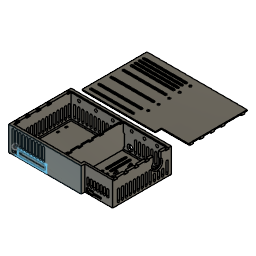
SKRMiniBox CNC (Autodesk Fusion 360 design; units mm, degrees)
part number: 2025-08-04-01-21-32-688
Autodesk Fusion 360 part; units mm, degrees
(part 1 of 2)
other "Base Mesh Feature1"
other "Modify1"
sketch "Sketch2" plane through (0, 0, 0) normal (0, 0, 1) x (1, 0, 0)
  line L0 (-173.9436, -72.9826) -> (-173.9268, 62.9979)
  line L1 (-173.9268, 62.9979) -> (52.0199, 63.0011)
  line L2 (52.0199, 63.0011) -> (52.0199, -64.6029)
  circle A0 centre (28.2811, 19.6527) radius 3.024
  circle A1 centre (-6.7121, 37.2637) radius 3.024
  circle A2 centre (28.2811, 19.6527) radius 3.024
  circle A3 centre (-9.3669, 5.4726) radius 3.024
  circle A4 centre (28.249, -42.7358) radius 3.024
  circle A5 centre (-36.2541, -58.894) radius 3.024
  line L3 (-180, 69) -> (58, 69)
  line L4 (58, 69) -> (58, -70.5015)
  line L5 (-8.0005, -79) -> (-180, -79)
  line L6 (-180, -79) -> (-180, 69)
  arc A6 (47.0198, 63.0011) -> (52.0199, 58.0011) centre (47.0199, 58.0011) ccw
  arc A7 (-168.9436, -72.9826) -> (-173.943, -67.982) centre (-168.943, -67.9826) ccw
  arc A8 (-173.9274, 57.9986) -> (-168.9275, 62.998) centre (-168.9274, 57.998) ccw
  line L7 (-163, 45) -> (-53, 45)
  line L8 (-53, 45) -> (-53, 40)
  line L9 (-53, 40) -> (-163, 40)
  line L10 (-163, 40) -> (-163, 45)
  line L11 (-163, 25) -> (-53, 25)
  line L12 (-53, 25) -> (-53, 20)
  line L13 (-53, 20) -> (-163, 20)
  line L14 (-163, 20) -> (-163, 25)
  line L15 (-163, 57) -> (-53, 57)
  line L16 (-53, 57) -> (-53, -23)
  line L17 (-53, -23) -> (-163, -23)
  line L18 (-163, -23) -> (-163, 57)
  line L19 (-163, -23) -> (-133, -23)
  line L20 (-133, -23) -> (-133, -73)
  line L21 (-133, -73) -> (-163, -73)
  line L22 (-163, -73) -> (-163, -23)
  line L23 (-13.9959, -72.9826) -> (-173.9436, -72.9826)
  line L24 (52.0199, -64.6029) -> (-14, -64.6029)
  line L25 (58, -70.5015) -> (-7.9998, -70.5015)
  line L26 (-13.9959, -72.9826) -> (-13.9959, -64.6029)
  line L27 (-11, -64.5017) -> (-11, -64.5)
  line L28 (-7.9998, -70.5015) -> (-8.0005, -79)
  arc A9 (52.0199, -59.6029) -> (47.0199, -64.6029) centre (47.0199, -59.6029) ccw
  line L29 (-53, 45) -> (-50, 45)
  line L30 (-50, 45) -> (-50, 40)
  line L31 (-50, 40) -> (-53, 40)
  line L32 (-53, 40) -> (-53, 45)
  line L33 (-163, 45) -> (-166, 45)
  line L34 (-166, 45) -> (-166, 40)
  line L35 (-166, 40) -> (-163, 40)
  line L36 (-163, 40) -> (-163, 45)
  line L37 (-53, 25) -> (-50, 25)
  line L38 (-50, 25) -> (-50, 20)
  line L39 (-50, 20) -> (-53, 20)
  line L40 (-53, 20) -> (-53, 25)
  line L41 (-163, 25) -> (-166, 25)
  line L42 (-166, 25) -> (-166, 20)
  line L43 (-166, 20) -> (-163, 20)
  line L44 (-163, 20) -> (-163, 25)
  line L45 (-133, -35) -> (-50, -35)
  line L46 (-50, -35) -> (-50, -40)
  line L47 (-50, -40) -> (-133, -40)
  line L48 (-133, -40) -> (-133, -35)
  line L49 (-163, -35) -> (-166, -35)
  line L50 (-166, -35) -> (-166, -40)
  line L51 (-166, -40) -> (-163, -40)
  line L52 (-163, -40) -> (-163, -35)
  line L53 (-133, -50) -> (-50, -50)
  line L54 (-50, -50) -> (-50, -55)
  line L55 (-50, -55) -> (-133, -55)
  line L56 (-133, -55) -> (-133, -50)
  line L57 (-163, -50) -> (-166, -50)
  line L58 (-166, -50) -> (-166, -55)
  line L59 (-166, -55) -> (-163, -55)
  line L60 (-163, -55) -> (-163, -50)
  line L61 (-133, -65) -> (-50, -65)
  line L62 (-50, -65) -> (-50, -70)
  line L63 (-50, -70) -> (-133, -70)
  line L64 (-133, -70) -> (-133, -65)
  line L65 (-163, -65) -> (-166, -65)
  line L66 (-166, -65) -> (-166, -70)
  line L67 (-166, -70) -> (-163, -70)
  line L68 (-163, -70) -> (-163, -65)
  dimension "d1" = 5
  dimension "d3" = 5
  dimension "d4" = 5
  dimension "d5" = 80
  dimension "d6" = 30
  dimension "d7" = 50
  dimension "d8" = 5
  constraint tangent L1 A6
  constraint tangent L2 A6
  constraint tangent L1 A8
  constraint tangent L0 A8
  constraint tangent L0 A7
  constraint horizontal L3
  constraint vertical L4
  constraint horizontal L5
  constraint vertical L6
  constraint coincident L2 A6.end
  constraint coincident L1 A6.start
  constraint coincident L0 A7.end
  constraint coincident L1 A8.end
  constraint coincident L0 A8.start
  constraint horizontal L7
  constraint vertical L8
  constraint horizontal L9
  constraint vertical L10
  constraint horizontal L11
  constraint vertical L12
  constraint horizontal L13
  constraint vertical L14
  constraint horizontal L15
  constraint vertical L16
  constraint horizontal L17
  constraint vertical L18
  constraint horizontal L19
  constraint vertical L20
  constraint horizontal L21
  constraint vertical L22
  constraint vertical L2
  constraint perpendicular L23 L26
  constraint coincident L24 L26.end
  constraint perpendicular L24 L26
  constraint tangent L2 A9
  constraint tangent L24 A9
  constraint coincident L24 A9.end
  constraint coincident L2 A9.start
  constraint tangent A7 L23
  constraint horizontal L29
  constraint vertical L30
  constraint horizontal L31
  constraint vertical L32
  constraint horizontal L33
  constraint vertical L34
  constraint horizontal L35
  constraint vertical L36
  constraint horizontal L37
  constraint vertical L38
  constraint horizontal L39
  constraint vertical L40
  constraint horizontal L41
  constraint vertical L42
  constraint horizontal L43
  constraint vertical L44
  constraint horizontal L45
  constraint vertical L46
  constraint horizontal L47
  constraint vertical L48
  constraint coincident L20 L45.start
  constraint horizontal L49
  constraint vertical L50
  constraint horizontal L51
  constraint vertical L52
  constraint coincident L22 L49.start
  constraint horizontal L53
  constraint vertical L54
  constraint horizontal L55
  constraint vertical L56
  constraint coincident L20 L53.start
  constraint horizontal L57
  constraint vertical L58
  constraint horizontal L59
  constraint vertical L60
  constraint coincident L22 L57.start
  constraint horizontal L61
  constraint vertical L62
  constraint horizontal L63
  constraint vertical L64
  constraint coincident L20 L61.start
  constraint horizontal L65
  constraint vertical L66
  constraint horizontal L67
  constraint vertical L68
  constraint coincident L22 L65.start
  measures "d1" radius of A6
  measures "d3" radius of A8
  measures "d4" radius of A7
  measures "d5" distance of L15.start L17.end
  measures "d6" distance of L17.end L19.end
  measures "d7" distance of L17.end L21.end
  measures "d8" radius of A9
extrude "Extrude1" add sketch "Sketch2" along normal blind 2 contours L0 A7 L23 L65 L66 L67 | L0 L1 L2 A6 A7 A8 L15 L16 L17 L18 L20 L22 L23 L24 L26 A9 L29 L30 L31 L33 L34 L35 L37 L38 L39 L41 L42 L43 L45 L46 L47 L49 L50 L51 L53 L54 L55 L57 L58 L59 L61 L62 L63 L65 | A7 L22 L23 L67 | L0 L1 A8 | A7 L22 L65 L67 L68 | A7 L65 L66 L67 | L20 L21 L22 L23 | L17 L19 L20 L22 L23 L48 L52 L56 L60 L64 L68 | L1 L2 A6 | L22 L57 L58 L59 L60 | L20 L61 L62 L63 L64 | L2 L24 A9 | L22 L49 L50 L51 L52 | L20 L53 L54 L55 L56 | L13 L16 L17 L18 L19 | L20 L45 L46 L47 L48 | L11 L12 L13 L14 L16 L18 L40 L44 | L14 L18 L41 L42 L43 L44 | L12 L16 L37 L38 L39 L40 | L9 L11 L16 L18 | L7 L8 L9 L10 L16 L18 L32 L36 | L10 L18 L33 L34 L35 L36 | L8 L16 L29 L30 L31 L32 | L7 L15 L16 L18 | A0 A2 | A1 | A3 | A4 | A5 | L3 L4 L5 L6 L25 L28 makes body 1
extrude "Extrude2" add sketch "Sketch2" along normal blind 46 separate body contours L3 L4 L5 L6 L25 L28 makes body 2
extrude "Extrude3" add sketch "Sketch2" along normal blind 7 separate body contours A0 A2 | A1 | A3 | A4 | A5 makes body 3 at (-6.3579, 5.1715, 4.6667) makes body 4 at (-3.7031, 36.9626, 4.6667) makes body 5 at (31.258, -43.0369, 4.6667) makes body 6 at (31.2901, 19.3516, 4.6667) makes body 7 at (-33.2451, -59.1951, 4.6667)
extrude "Extrude4" add sketch "Sketch2" along normal blind 20 contours L11 L12 L13 L14 L16 L18 L40 L44 | L7 L8 L9 L10 L16 L18 L32 L36 bodies 1
sketch "Sketch3" plane through (0, 20, 0) normal (0, -1, 0) x (1, 0, 0)
  line L0 (-163, 2) -> (-53, 2)
  line L1 (-53, 2) -> (-53, 20)
  line L2 (-53, 20) -> (-163, 20)
  line L3 (-163, 20) -> (-163, 2)
  circle A0 centre (-68, 19) radius 12.5
  dimension "d17" = 25
  measures "d17" diameter of A0
extrude "Extrude5" cut sketch "Sketch3" against normal blind 28 contours L2 A0 picked at (-64.6798, 14.1417) bodies 1
extrude "Extrude6" cut sketch "Sketch2" along normal blind 4 contours A7 L22 L65 L67 L68 | A7 L65 L66 L67 | L22 L57 L58 L59 L60 | L20 L61 L62 L63 L64 | L22 L49 L50 L51 L52 | L20 L53 L54 L55 L56 | L20 L45 L46 L47 L48 | L14 L18 L41 L42 L43 L44 | L12 L16 L37 L38 L39 L40 | L10 L18 L33 L34 L35 L36 | L8 L16 L29 L30 L31 L32 bodies 1
sketch "Sketch4" plane through (0, -64.6029, 0) normal (0, 1, 0) x (-1, 0, 0)
  line L0 (-52.0199, 0) -> (13.9959, 0)
  line L1 (13.9959, 0) -> (13.9959, 46)
  line L2 (13.9959, 46) -> (-52.0199, 46)
  line L3 (-52.0199, 46) -> (-52.0199, 0)
  line L4 (-11, 14) -> (3, 14)
  line L5 (3, 14) -> (3, 6)
  line L6 (3, 6) -> (-11, 6)
  line L7 (-11, 6) -> (-11, 14)
  line L8 (-30.5509, 11) -> (-12.8347, 11)
  line L9 (-12.8347, 11) -> (-12.8347, 8)
  line L10 (-12.8347, 8) -> (-30.5509, 8)
  line L11 (-30.5509, 8) -> (-30.5509, 11)
  constraint horizontal L4
  constraint vertical L5
  constraint horizontal L6
  constraint vertical L7
  constraint horizontal L8
  constraint vertical L9
  constraint horizontal L10
  constraint vertical L11
extrude "Extrude7" cut sketch "Sketch4" against normal blind 10 contours L4 L5 L6 L7 | L8 L9 L10 L11 bodies 2
sketch "Sketch5" plane through (58, 0, 0) normal (1, 0, 0) x (0, 1, 0)
  line L0 (-70.5015, 0) -> (69, 0)
  line L1 (69, 0) -> (69, 46)
  line L2 (69, 46) -> (-70.5015, 46)
  line L3 (-70.5015, 46) -> (-70.5015, 0)
  circle A0 centre (35, 40) radius 11
extrude "Extrude8" cut sketch "Sketch5" against normal blind 9 contours L2 A0 picked at (37.7089, 36.3656) bodies 2
sketch "Sketch6" plane through (0, 69, 0) normal (0, 1, 0) x (-1, 0, 0)
  line L0 (-58, 0) -> (180, 0)
  line L1 (180, 0) -> (180, 46)
  line L2 (180, 46) -> (-58, 46)
  line L3 (-58, 46) -> (-58, 0)
  circle A0 centre (34, 14) radius 5
extrude "Extrude9" cut sketch "Sketch6" against normal blind 8 contours A0 bodies 2
extrude "Extrude10" add 1 faces at (-177.9812, -27.6609, 46) along direction (0, 0, 1) blind 15 on bodies 2 bodies 2
sketch "Sketch7" plane through (58, 0, 0) normal (1, 0, 0) x (0, 1, 0)
  line L0 (25.7805, 61) -> (-70.5015, 61)
  line L1 (-70.5015, 61) -> (-70.5015, 0)
  line L2 (-70.5015, 0) -> (69, 0)
  line L3 (69, 0) -> (69, 61)
  arc A0 (25.7805, 46) -> (44.2195, 46) centre (35, 40) ccw
  line L4 (62, 43) -> (64, 40)
  line L5 (64, 40) -> (55, 40)
  line L6 (55, 40) -> (57, 43)
  line L7 (3, 61) -> (5, 58)
  line L8 (5, 58) -> (-5, 58)
  line L9 (-5, 58) -> (-3, 61)
  line L10 (-22, 61) -> (-20, 58)
  line L11 (-20, 58) -> (-30, 58)
  line L12 (-30, 58) -> (-28, 61)
  line L13 (-47, 61) -> (-45, 58)
  line L14 (-45, 58) -> (-55, 58)
  line L15 (-55, 58) -> (-53, 61)
  line L16 (-72, 61) -> (-70, 58)
  line L17 (-70, 58) -> (-80, 58)
  line L18 (-80, 58) -> (-78, 61)
  line L19 (242, 43) -> (244, 40)
  line L20 (162, 40) -> (164, 43)
  line L21 (147, 40) -> (137, 40)
  line L22 (137, 40) -> (139, 43)
  line L23 (187, 40) -> (189, 43)
  line L24 (195, 43) -> (197, 40)
  line L25 (112, 40) -> (114, 43)
  line L26 (197, 40) -> (187, 40)
  line L27 (172, 40) -> (162, 40)
  line L28 (235, 40) -> (237, 43)
  line L29 (122, 40) -> (112, 40)
  line L30 (120, 43) -> (122, 40)
  line L31 (145, 43) -> (147, 40)
  line L32 (170, 43) -> (172, 40)
  line L33 (249, 43) -> (225.583, 43)
  line L34 (244, 40) -> (235, 40)
  line L35 (204.417, 43) -> (109.4985, 43)
  line L36 (225.583, 43) -> (204.417, 43)
  line L37 (243.95, 40) -> (241.95, 43)
  line L38 (243.95, 40.05) -> (235, 40.05)
  line L39 (235.05, 40) -> (237.05, 43)
  line L40 (194.9089, 43) -> (196.9089, 40)
  line L41 (196.9, 40.1) -> (187.0667, 40.1)
  line L42 (187.1, 40) -> (189.1, 43)
  line L43 (169.9, 43) -> (171.9, 40)
  line L44 (171.9, 40.1) -> (162.0667, 40.1)
  line L45 (162.1, 40) -> (164.1, 43)
  line L46 (144.9, 43) -> (146.9, 40)
  line L47 (146.9, 40.1) -> (137.0667, 40.1)
  line L48 (137.1, 40) -> (139.1, 43)
  line L49 (119.9, 43) -> (121.9, 40)
  line L50 (121.9, 40.1) -> (112.0667, 40.1)
  line L51 (112.1, 40) -> (114.1, 43)
  line L52 (109.4985, 43) -> (109.4985, 45.5)
  line L53 (109.4985, 45.5) -> (249, 45.5)
  line L54 (249, 43) -> (249, 45.5)
  line L55 (25.7805, 46) -> (25.7805, 61)
  line L56 (69, 61) -> (44.2195, 61)
  line L57 (44.2195, 61) -> (44.2195, 46)
  dimension "d30" = 10
  dimension "d33" = 10
  dimension "d34" = 2.5
  constraint coincident L0 L7.start
  constraint parallel L4 L7
  constraint parallel L0 L8
  constraint coincident L0 L9.end
  constraint coincident L0 L10.start
  constraint parallel L8 L11
  constraint parallel L9 L12
  constraint coincident L0 L13.start
  constraint parallel L10 L13
  constraint parallel L0 L14
  constraint coincident L0 L15.end
  constraint parallel L12 L15
  constraint coincident L0 L16.start
  constraint parallel L13 L16
  constraint parallel L0 L17
  constraint coincident L0 L18.end
  constraint parallel L15 L18
  constraint coincident L19.start L33
  constraint parallel L33 L34
  constraint coincident L28.end L33
  constraint coincident L24.start L35
  constraint parallel L19 L24
  constraint parallel L26 L35
  constraint coincident L23.end L35
  constraint coincident L32.start L35
  constraint parallel L26 L27
  constraint parallel L20 L23
  constraint coincident L31.start L35
  constraint parallel L31 L32
  constraint parallel L21 L35
  constraint coincident L22.end L35
  constraint parallel L20 L22
  constraint coincident L30.start L35
  constraint parallel L30 L31
  constraint parallel L29 L35
  constraint coincident L25.end L35
  constraint parallel L22 L25
  constraint parallel L35 L36
  constraint coincident L34 L37.start
  constraint coincident L33 L37.end
  constraint parallel L19 L37
  constraint parallel L34 L38
  constraint coincident L34 L39.start
  constraint coincident L33 L39.end
  constraint parallel L28 L39
  constraint coincident L26 L40.end
  constraint parallel L24 L40
  constraint coincident L23 L41.end
  constraint parallel L26 L41
  constraint coincident L26 L42.start
  constraint coincident L35 L42.end
  constraint parallel L23 L42
  constraint coincident L35 L43.start
  constraint coincident L27 L43.end
  constraint parallel L32 L43
  constraint coincident L20 L44.end
  constraint parallel L27 L44
  constraint coincident L27 L45.start
  constraint coincident L35 L45.end
  constraint parallel L20 L45
  constraint coincident L21 L46.end
  constraint parallel L31 L46
  constraint coincident L22 L47.end
  constraint parallel L21 L47
  constraint coincident L21 L48.start
  constraint coincident L35 L48.end
  constraint parallel L22 L48
  constraint coincident L35 L49.start
  constraint coincident L29 L49.end
  constraint parallel L30 L49
  constraint coincident L25 L50.end
  constraint parallel L29 L50
  constraint coincident L29 L51.start
  constraint coincident L35 L51.end
  constraint parallel L25 L51
  constraint perpendicular L35 L52
  constraint perpendicular L52 L53
  constraint perpendicular L53 L54
  measures "d30" distance of L10.end L11.end
  measures "d33" distance of L20.start L27.start
  measures "d34" distance of L35.end L52.end
other "Modify2"
extrude "Extrude12" add sketch "Sketch7" against normal blind 156 separate body contours L33 L35 L36 L52 L53 L54 | L33 L37 L38 L39 | L35 L49 L50 L51 | L35 L40 L41 L42 | L35 L46 L47 L48 | L35 L43 L44 L45 makes body 8
sketch "Sketch8" plane through (0, 0, 43) normal (0, 0, -1) x (1, 0, 0)
  line L0 (58, -237.05) -> (58, -194.9089)
  line L1 (58, -194.9089) -> (-98, -194.9089)
  line L2 (-98, -194.9089) -> (-98, -237.05)
  line L3 (-98, -237.05) -> (58, -237.05)
  circle A0 centre (-58, -230.0227) radius 2.75
  circle A1 centre (-58, -204.6724) radius 2.75
  dimension "d37" = 5.5
  dimension "d153" = 40
  dimension "d154" = 40
  constraint equal A0 A1
  measures "d37" diameter of A0
  measures "d153" distance of L2 A1.centre
  measures "d154" distance of L2 A0.centre
sketch "Sketch9" plane through (0, 0, 43) normal (0, 0, -1) x (1, 0, 0)
  line L0 (58, -189.1) -> (58, -169.9)
  line L1 (58, -169.9) -> (-98, -169.9)
  line L2 (-98, -169.9) -> (-98, -189.1)
  line L3 (-98, -189.1) -> (58, -189.1)
  circle A0 centre (-58, -179.8487) radius 2.75
  dimension "d40" = 5.5
  dimension "d152" = 40
  measures "d40" diameter of A0
  measures "d152" distance of L2 A0.centre
sketch "Sketch10" plane through (0, 0, 43) normal (0, 0, -1) x (1, 0, 0)
  line L0 (58, -164.1) -> (58, -144.9)
  line L1 (58, -144.9) -> (-98, -144.9)
  line L2 (-98, -144.9) -> (-98, -164.1)
  line L3 (-98, -164.1) -> (58, -164.1)
  circle A0 centre (-58, -154.7263) radius 2.75
  dimension "d42" = 5.5
  dimension "d151" = 40
  measures "d42" diameter of A0
  measures "d151" distance of L2 A0.centre
sketch "Sketch11" plane through (0, 0, 43) normal (0, 0, -1) x (1, 0, 0)
  line L0 (58, -139.1) -> (58, -119.9)
  line L1 (58, -119.9) -> (-98, -119.9)
  line L2 (-98, -119.9) -> (-98, -139.1)
  line L3 (-98, -139.1) -> (58, -139.1)
  circle A0 centre (-58, -129.8013) radius 2.75
  dimension "d44" = 5.5
  dimension "d150" = 40
  measures "d44" diameter of A0
  measures "d150" distance of L2 A0.centre
extrude "Extrude13" cut sketch "Sketch10" sketch "Sketch8" sketch "Sketch9" sketch "Sketch11" against normal blind 5 contours A0 of sketch 2 contours A0 | A1 of sketch 3 contours A0 of sketch 4 contours A0 bodies 8
sketch "Sketch12" plane through (0, -79, 0) normal (0, -1, 0) x (1, 0, 0)
  line L0 (-8.0005, 61) -> (-180, 61)
  line L1 (-180, 61) -> (-180, 0)
  line L2 (-180, 0) -> (-8.0005, 0)
  line L3 (-8.0005, 0) -> (-8.0005, 61)
  line L4 (-167, 88.1773) -> (-167, 10)
  line L5 (-172, 10) -> (-172, 88.1773)
  arc A0 (-167, 88.1773) -> (-172, 88.1773) centre (-169.5, 88.1773) ccw
  arc A1 (-172, 10) -> (-167, 10) centre (-169.5, 10) ccw
  line L6 (-159, 88.1773) -> (-159, 10)
  arc A2 (-159, 88.1773) -> (-164, 88.1773) centre (-161.5, 88.1773) ccw
  line L7 (-164, 10) -> (-164, 88.1773)
  arc A3 (-164, 10) -> (-159, 10) centre (-161.5, 10) ccw
  line L8 (-151, 88.1773) -> (-151, 10)
  arc A4 (-151, 88.1773) -> (-156, 88.1773) centre (-153.5, 88.1773) ccw
  line L9 (-156, 10) -> (-156, 88.1773)
  arc A5 (-156, 10) -> (-151, 10) centre (-153.5, 10) ccw
  line L10 (-143, 88.1773) -> (-143, 10)
  arc A6 (-143, 88.1773) -> (-148, 88.1773) centre (-145.5, 88.1773) ccw
  line L11 (-148, 10) -> (-148, 88.1773)
  arc A7 (-148, 10) -> (-143, 10) centre (-145.5, 10) ccw
  line L12 (-135, 88.1773) -> (-135, 10)
  arc A8 (-135, 88.1773) -> (-140, 88.1773) centre (-137.5, 88.1773) ccw
  line L13 (-140, 10) -> (-140, 88.1773)
  arc A9 (-140, 10) -> (-135, 10) centre (-137.5, 10) ccw
  line L14 (-127, 88.1773) -> (-127, 10)
  arc A10 (-127, 88.1773) -> (-132, 88.1773) centre (-129.5, 88.1773) ccw
  line L15 (-132, 10) -> (-132, 88.1773)
  arc A11 (-132, 10) -> (-127, 10) centre (-129.5, 10) ccw
  line L16 (-119, 88.1773) -> (-119, 10)
  arc A12 (-119, 88.1773) -> (-124, 88.1773) centre (-121.5, 88.1773) ccw
  line L17 (-124, 10) -> (-124, 88.1773)
  arc A13 (-124, 10) -> (-119, 10) centre (-121.5, 10) ccw
  line L18 (-111, 88.1773) -> (-111, 10)
  arc A14 (-111, 88.1773) -> (-116, 88.1773) centre (-113.5, 88.1773) ccw
  line L19 (-116, 10) -> (-116, 88.1773)
  arc A15 (-116, 10) -> (-111, 10) centre (-113.5, 10) ccw
  line L20 (-103, 88.1773) -> (-103, 10)
  arc A16 (-103, 88.1773) -> (-108, 88.1773) centre (-105.5, 88.1773) ccw
  line L21 (-108, 10) -> (-108, 88.1773)
  arc A17 (-108, 10) -> (-103, 10) centre (-105.5, 10) ccw
  line L22 (-95, 88.1773) -> (-95, 10)
  arc A18 (-95, 88.1773) -> (-100, 88.1773) centre (-97.5, 88.1773) ccw
  line L23 (-100, 10) -> (-100, 88.1773)
  arc A19 (-100, 10) -> (-95, 10) centre (-97.5, 10) ccw
  dimension "d48" = 5
  dimension "d51" = 72
  dimension "d52" = 0
  constraint vertical L4
  constraint vertical L5
  measures "d48" diameter of A0
extrude "Extrude14" cut sketch "Sketch12" against normal blind 10 contours L0 L22 L23 A19 | L0 L22 A18 L23 | L0 L20 L21 A17 | L0 L20 A16 L21 | L0 L4 L5 A0 | L0 L4 L5 A1 | L0 L18 L19 A15 | L0 L18 A14 L19 | L0 L6 A2 L7 | L0 L6 L7 A3 | L0 L16 L17 A13 | L0 L16 A12 L17 | L0 L8 A4 L9 | L0 L8 L9 A5 | L0 L14 L15 A11 | L0 L14 A10 L15 | L0 L10 A6 L11 | L0 L10 L11 A7 | L0 L12 L13 A9 | L0 L12 A8 L13 bodies 2
sketch "Sketch13" plane through (0, -70.5015, 0) normal (0, -1, 0) x (1, 0, 0)
  line L0 (-7.9998, 61) -> (-7.9998, 0)
  line L1 (-7.9998, 0) -> (58, 0)
  line L2 (58, 0) -> (58, 61)
  line L3 (12.8347, 8) -> (12.8347, 11)
  line L4 (12.8347, 11) -> (30.5509, 11)
  line L5 (30.5509, 11) -> (30.5509, 8)
  line L6 (30.5509, 8) -> (12.8347, 8)
  line L7 (-3, 6) -> (-3, 14)
  line L8 (-3, 14) -> (11, 14)
  line L9 (11, 14) -> (11, 6)
  line L10 (11, 6) -> (-3, 6)
  line L11 (2, 35) -> (2, 21)
  arc A0 (2, 35) -> (-3, 35) centre (-0.5, 35) ccw
  line L12 (-3, 21) -> (-3, 35)
  arc A1 (-3, 21) -> (2, 21) centre (-0.5, 21) ccw
  line L13 (4.8333, 21) -> (4.8333, 35)
  arc A2 (9.8333, 35) -> (4.8333, 35) centre (7.3333, 35) ccw
  line L14 (9.8333, 35) -> (9.8333, 21)
  arc A3 (4.8333, 21) -> (9.8333, 21) centre (7.3333, 21) ccw
  line L15 (12.6667, 21) -> (12.6667, 35)
  arc A4 (17.6667, 35) -> (12.6667, 35) centre (15.1667, 35) ccw
  line L16 (17.6667, 35) -> (17.6667, 21)
  arc A5 (12.6667, 21) -> (17.6667, 21) centre (15.1667, 21) ccw
  line L17 (20.5, 21) -> (20.5, 35)
  arc A6 (25.5, 35) -> (20.5, 35) centre (23, 35) ccw
  line L18 (25.5, 35) -> (25.5, 21)
  arc A7 (20.5, 21) -> (25.5, 21) centre (23, 21) ccw
  line L19 (28.3333, 21) -> (28.3333, 35)
  arc A8 (33.3333, 35) -> (28.3333, 35) centre (30.8333, 35) ccw
  line L20 (33.3333, 35) -> (33.3333, 21)
  arc A9 (28.3333, 21) -> (33.3333, 21) centre (30.8333, 21) ccw
  line L21 (36.1667, 21) -> (36.1667, 35)
  arc A10 (41.1667, 35) -> (36.1667, 35) centre (38.6667, 35) ccw
  line L22 (41.1667, 35) -> (41.1667, 21)
  arc A11 (36.1667, 21) -> (41.1667, 21) centre (38.6667, 21) ccw
  line L23 (44, 21) -> (44, 35)
  arc A12 (49, 35) -> (44, 35) centre (46.5, 35) ccw
  line L24 (49, 35) -> (49, 21)
  arc A13 (44, 21) -> (49, 21) centre (46.5, 21) ccw
  line L25 (58, 61) -> (-7.9998, 61)
  dimension "d57" = 47
  dimension "d58" = 0
extrude "Extrude15" cut sketch "Sketch13" against normal blind 7 contours L11 A0 L12 A1 | L13 A2 L14 A3 | L15 A4 L16 A5 | L17 A6 L18 A7 | L19 A8 L20 A9 | L21 A10 L22 A11 | L23 A12 L24 A13 bodies 2
sketch "Sketch14" plane through (-180, 0, 0) normal (-1, 0, 0) x (0, -1, 0)
  line L0 (79, 61) -> (-69, 61)
  line L1 (-69, 61) -> (-69, 0)
  line L2 (-69, 0) -> (79, 0)
  line L3 (79, 0) -> (79, 61)
  line L4 (-56, 35) -> (-56, 10)
  arc A0 (-56, 35) -> (-61, 35) centre (-58.5, 35) ccw
  line L5 (-61, 10) -> (-61, 35)
  arc A1 (-61, 10) -> (-56, 10) centre (-58.5, 10) ccw
  line L6 (-47.0714, 35) -> (-47.0714, 10)
  arc A2 (-47.0714, 35) -> (-52.0714, 35) centre (-49.5714, 35) ccw
  line L7 (-52.0714, 10) -> (-52.0714, 35)
  arc A3 (-52.0714, 10) -> (-47.0714, 10) centre (-49.5714, 10) ccw
  line L8 (-38.1429, 35) -> (-38.1429, 10)
  arc A4 (-38.1429, 35) -> (-43.1429, 35) centre (-40.6429, 35) ccw
  line L9 (-43.1429, 10) -> (-43.1429, 35)
  arc A5 (-43.1429, 10) -> (-38.1429, 10) centre (-40.6429, 10) ccw
  line L10 (-29.2143, 35) -> (-29.2143, 10)
  arc A6 (-29.2143, 35) -> (-34.2143, 35) centre (-31.7143, 35) ccw
  line L11 (-34.2143, 10) -> (-34.2143, 35)
  arc A7 (-34.2143, 10) -> (-29.2143, 10) centre (-31.7143, 10) ccw
  line L12 (-20.2857, 35) -> (-20.2857, 10)
  arc A8 (-20.2857, 35) -> (-25.2857, 35) centre (-22.7857, 35) ccw
  line L13 (-25.2857, 10) -> (-25.2857, 35)
  arc A9 (-25.2857, 10) -> (-20.2857, 10) centre (-22.7857, 10) ccw
  line L14 (-11.3571, 35) -> (-11.3571, 10)
  arc A10 (-11.3571, 35) -> (-16.3571, 35) centre (-13.8571, 35) ccw
  line L15 (-16.3571, 10) -> (-16.3571, 35)
  arc A11 (-16.3571, 10) -> (-11.3571, 10) centre (-13.8571, 10) ccw
  line L16 (-2.4286, 35) -> (-2.4286, 10)
  arc A12 (-2.4286, 35) -> (-7.4286, 35) centre (-4.9286, 35) ccw
  line L17 (-7.4286, 10) -> (-7.4286, 35)
  arc A13 (-7.4286, 10) -> (-2.4286, 10) centre (-4.9286, 10) ccw
  line L18 (6.5, 35) -> (6.5, 10)
  arc A14 (6.5, 35) -> (1.5, 35) centre (4, 35) ccw
  line L19 (1.5, 10) -> (1.5, 35)
  arc A15 (1.5, 10) -> (6.5, 10) centre (4, 10) ccw
  line L20 (15.4286, 35) -> (15.4286, 10)
  arc A16 (15.4286, 35) -> (10.4286, 35) centre (12.9286, 35) ccw
  line L21 (10.4286, 10) -> (10.4286, 35)
  arc A17 (10.4286, 10) -> (15.4286, 10) centre (12.9286, 10) ccw
  line L22 (24.3571, 35) -> (24.3571, 10)
  arc A18 (24.3571, 35) -> (19.3571, 35) centre (21.8571, 35) ccw
  line L23 (19.3571, 10) -> (19.3571, 35)
  arc A19 (19.3571, 10) -> (24.3571, 10) centre (21.8571, 10) ccw
  line L24 (33.2857, 35) -> (33.2857, 10)
  arc A20 (33.2857, 35) -> (28.2857, 35) centre (30.7857, 35) ccw
  line L25 (28.2857, 10) -> (28.2857, 35)
  arc A21 (28.2857, 10) -> (33.2857, 10) centre (30.7857, 10) ccw
  line L26 (42.2143, 35) -> (42.2143, 10)
  arc A22 (42.2143, 35) -> (37.2143, 35) centre (39.7143, 35) ccw
  line L27 (37.2143, 10) -> (37.2143, 35)
  arc A23 (37.2143, 10) -> (42.2143, 10) centre (39.7143, 10) ccw
  line L28 (51.1429, 35) -> (51.1429, 10)
  arc A24 (51.1429, 35) -> (46.1429, 35) centre (48.6429, 35) ccw
  line L29 (46.1429, 10) -> (46.1429, 35)
  arc A25 (46.1429, 10) -> (51.1429, 10) centre (48.6429, 10) ccw
  line L30 (60.0714, 35) -> (60.0714, 10)
  arc A26 (60.0714, 35) -> (55.0714, 35) centre (57.5714, 35) ccw
  line L31 (55.0714, 10) -> (55.0714, 35)
  arc A27 (55.0714, 10) -> (60.0714, 10) centre (57.5714, 10) ccw
  line L32 (69, 35) -> (69, 10)
  arc A28 (69, 35) -> (64, 35) centre (66.5, 35) ccw
  line L33 (64, 10) -> (64, 35)
  arc A29 (64, 10) -> (69, 10) centre (66.5, 10) ccw
  dimension "d63" = 125
  dimension "d64" = 0
extrude "Extrude16" cut sketch "Sketch14" against normal blind 10 contours L4 A0 L5 A1 | L6 A2 L7 A3 | L8 A4 L9 A5 | L10 A6 L11 A7 | L12 A8 L13 A9 | L14 A10 L15 A11 | L16 A12 L17 A13 | L18 A14 L19 A15 | L20 A16 L21 A17 | L22 A18 L23 A19 | L24 A20 L25 A21 | L26 A22 L27 A23 | L28 A24 L29 A25 | L30 A26 L31 A27 | L32 A28 L33 A29 bodies 2
sketch "Sketch15" plane through (0, 69, 0) normal (0, 1, 0) x (-1, 0, 0)
  line L0 (180, 61) -> (-58, 61)
  line L1 (-58, 61) -> (-58, 0)
  line L2 (-58, 0) -> (180, 0)
  line L3 (180, 0) -> (180, 61)
  circle A0 centre (34, 14) radius 5
  line L4 (-44, 35) -> (-44, 10)
  arc A1 (-44, 35) -> (-49, 35) centre (-46.5, 35) ccw
  line L5 (-49, 10) -> (-49, 35)
  arc A2 (-49, 10) -> (-44, 10) centre (-46.5, 10) ccw
  line L6 (-34.3571, 35) -> (-34.3571, 10)
  arc A3 (-34.3571, 35) -> (-39.3571, 35) centre (-36.8571, 35) ccw
  line L7 (-39.3571, 10) -> (-39.3571, 35)
  arc A4 (-39.3571, 10) -> (-34.3571, 10) centre (-36.8571, 10) ccw
  line L8 (-24.7143, 35) -> (-24.7143, 10)
  arc A5 (-24.7143, 35) -> (-29.7143, 35) centre (-27.2143, 35) ccw
  line L9 (-29.7143, 10) -> (-29.7143, 35)
  arc A6 (-29.7143, 10) -> (-24.7143, 10) centre (-27.2143, 10) ccw
  line L10 (-15.0714, 35) -> (-15.0714, 10)
  arc A7 (-15.0714, 35) -> (-20.0714, 35) centre (-17.5714, 35) ccw
  line L11 (-20.0714, 10) -> (-20.0714, 35)
  arc A8 (-20.0714, 10) -> (-15.0714, 10) centre (-17.5714, 10) ccw
  line L12 (-5.4286, 35) -> (-5.4286, 10)
  arc A9 (-5.4286, 35) -> (-10.4286, 35) centre (-7.9286, 35) ccw
  line L13 (-10.4286, 10) -> (-10.4286, 35)
  arc A10 (-10.4286, 10) -> (-5.4286, 10) centre (-7.9286, 10) ccw
  line L14 (4.2143, 35) -> (4.2143, 10)
  arc A11 (4.2143, 35) -> (-0.7857, 35) centre (1.7143, 35) ccw
  line L15 (-0.7857, 10) -> (-0.7857, 35)
  arc A12 (-0.7857, 10) -> (4.2143, 10) centre (1.7143, 10) ccw
  line L16 (13.8571, 35) -> (13.8571, 10)
  arc A13 (13.8571, 35) -> (8.8571, 35) centre (11.3571, 35) ccw
  line L17 (8.8571, 10) -> (8.8571, 35)
  arc A14 (8.8571, 10) -> (13.8571, 10) centre (11.3571, 10) ccw
  line L18 (23.5, 35) -> (23.5, 10)
  arc A15 (23.5, 35) -> (18.5, 35) centre (21, 35) ccw
  line L19 (18.5, 10) -> (18.5, 35)
  arc A16 (18.5, 10) -> (23.5, 10) centre (21, 10) ccw
  line L20 (52.4286, 35) -> (52.4286, 10)
  arc A17 (52.4286, 35) -> (47.4286, 35) centre (49.9286, 35) ccw
  line L21 (47.4286, 10) -> (47.4286, 35)
  arc A18 (47.4286, 10) -> (52.4286, 10) centre (49.9286, 10) ccw
  line L22 (62.0714, 35) -> (62.0714, 10)
  arc A19 (62.0714, 35) -> (57.0714, 35) centre (59.5714, 35) ccw
  line L23 (57.0714, 10) -> (57.0714, 35)
  arc A20 (57.0714, 10) -> (62.0714, 10) centre (59.5714, 10) ccw
  line L24 (71.7143, 35) -> (71.7143, 10)
  arc A21 (71.7143, 35) -> (66.7143, 35) centre (69.2143, 35) ccw
  line L25 (66.7143, 10) -> (66.7143, 35)
  arc A22 (66.7143, 10) -> (71.7143, 10) centre (69.2143, 10) ccw
  line L26 (81.3571, 35) -> (81.3571, 10)
  arc A23 (81.3571, 35) -> (76.3571, 35) centre (78.8571, 35) ccw
  line L27 (76.3571, 10) -> (76.3571, 35)
  arc A24 (76.3571, 10) -> (81.3571, 10) centre (78.8571, 10) ccw
  line L28 (91, 35) -> (91, 10)
  arc A25 (91, 35) -> (86, 35) centre (88.5, 35) ccw
  line L29 (86, 10) -> (86, 35)
  arc A26 (86, 10) -> (91, 10) centre (88.5, 10) ccw
extrude "Extrude17" cut sketch "Sketch15" against normal blind 10 contours L4 A1 L5 A2 | L6 A3 L7 A4 | L8 A5 L9 A6 | L10 A7 L11 A8 | L12 A9 L13 A10 | L14 A11 L15 A12 | L16 A13 L17 A14 | L18 A15 L19 A16 | L20 A17 L21 A18 | L22 A19 L23 A20 | L24 A21 L25 A22 | L26 A23 L27 A24 | L28 A25 L29 A26 bodies 2
sketch "Sketch16" plane through (58, 0, 0) normal (1, 0, 0) x (0, 1, 0)
  line L0 (69, 61) -> (44.2195, 61)
  line L1 (25.7805, 61) -> (-70.5015, 61)
  line L2 (-70.5015, 61) -> (-70.5015, 0)
  line L3 (-70.5015, 0) -> (69, 0)
  line L4 (69, 0) -> (69, 61)
  arc A0 (25.7805, 46) -> (44.2195, 46) centre (35, 40) ccw
  line L5 (-54, 35) -> (-54, 10)
  arc A1 (-54, 35) -> (-59, 35) centre (-56.5, 35) ccw
  line L6 (-59, 10) -> (-59, 35)
  arc A2 (-59, 10) -> (-54, 10) centre (-56.5, 10) ccw
  line L7 (-44.625, 35) -> (-44.625, 10)
  arc A3 (-44.625, 35) -> (-49.625, 35) centre (-47.125, 35) ccw
  line L8 (-49.625, 10) -> (-49.625, 35)
  arc A4 (-49.625, 10) -> (-44.625, 10) centre (-47.125, 10) ccw
  line L9 (-35.25, 35) -> (-35.25, 10)
  arc A5 (-35.25, 35) -> (-40.25, 35) centre (-37.75, 35) ccw
  line L10 (-40.25, 10) -> (-40.25, 35)
  arc A6 (-40.25, 10) -> (-35.25, 10) centre (-37.75, 10) ccw
  line L11 (-25.875, 35) -> (-25.875, 10)
  arc A7 (-25.875, 35) -> (-30.875, 35) centre (-28.375, 35) ccw
  line L12 (-30.875, 10) -> (-30.875, 35)
  arc A8 (-30.875, 10) -> (-25.875, 10) centre (-28.375, 10) ccw
  line L13 (-16.5, 35) -> (-16.5, 10)
  arc A9 (-16.5, 35) -> (-21.5, 35) centre (-19, 35) ccw
  line L14 (-21.5, 10) -> (-21.5, 35)
  arc A10 (-21.5, 10) -> (-16.5, 10) centre (-19, 10) ccw
  line L15 (-7.125, 35) -> (-7.125, 10)
  arc A11 (-7.125, 35) -> (-12.125, 35) centre (-9.625, 35) ccw
  line L16 (-12.125, 10) -> (-12.125, 35)
  arc A12 (-12.125, 10) -> (-7.125, 10) centre (-9.625, 10) ccw
  line L17 (2.25, 35) -> (2.25, 10)
  arc A13 (2.25, 35) -> (-2.75, 35) centre (-0.25, 35) ccw
  line L18 (-2.75, 10) -> (-2.75, 35)
  arc A14 (-2.75, 10) -> (2.25, 10) centre (-0.25, 10) ccw
  line L19 (11.625, 35) -> (11.625, 10)
  arc A15 (11.625, 35) -> (6.625, 35) centre (9.125, 35) ccw
  line L20 (6.625, 10) -> (6.625, 35)
  arc A16 (6.625, 10) -> (11.625, 10) centre (9.125, 10) ccw
  line L21 (21, 35) -> (21, 10)
  arc A17 (21, 35) -> (16, 35) centre (18.5, 35) ccw
  line L22 (16, 10) -> (16, 35)
  arc A18 (16, 10) -> (21, 10) centre (18.5, 10) ccw
  line L23 (-39, 35) -> (-39, 10)
  arc A19 (-39, 35) -> (-44, 35) centre (-41.5, 35) ccw
  line L24 (-44, 10) -> (-44, 35)
  arc A20 (-44, 10) -> (-39, 10) centre (-41.5, 10) ccw
  line L25 (31, 23) -> (31, 10)
  arc A21 (31, 23) -> (26, 23) centre (28.5, 23) ccw
  line L26 (26, 10) -> (26, 23)
  arc A22 (26, 10) -> (31, 10) centre (28.5, 10) ccw
  line L27 (61, 35) -> (61, 10)
  arc A23 (61, 35) -> (56, 35) centre (58.5, 35) ccw
  line L28 (56, 10) -> (56, 35)
  arc A24 (56, 10) -> (61, 10) centre (58.5, 10) ccw
  line L29 (41, 23) -> (41, 10)
  arc A25 (41, 23) -> (36, 23) centre (38.5, 23) ccw
  line L30 (36, 10) -> (36, 23)
  arc A26 (36, 10) -> (41, 10) centre (38.5, 10) ccw
  line L31 (51, 23) -> (51, 10)
  arc A27 (51, 23) -> (46, 23) centre (48.5, 23) ccw
  line L32 (46, 10) -> (46, 23)
  arc A28 (46, 10) -> (51, 10) centre (48.5, 10) ccw
  line L33 (44.2195, 61) -> (44.2195, 46)
  line L34 (25.7805, 46) -> (25.7805, 61)
  dimension "d75" = 75
  dimension "d76" = 0
  dimension "d79" = 20
  dimension "d80" = 0
extrude "Extrude18" cut sketch "Sketch16" against normal blind 10 contours L5 A1 L6 A2 | L7 A3 L8 A4 | L9 A5 A6 L23 A19 A20 | A5 L10 A6 L23 A19 A20 | L11 A7 L12 A8 | L13 A9 L14 A10 | L15 A11 L16 A12 | L17 A13 L18 A14 | L19 A15 L20 A16 | L21 A17 L22 A18 | L25 A21 L26 A22 | L27 A23 L28 A24 | L29 A25 L30 A26 | L31 A27 L32 A28 bodies 2
sketch "Sketch17" plane through (0, 0, 0) normal (0, 0, 1) x (1, 0, 0)
  line L0 (-29, 50) -> (-29, 5)
  arc A0 (-29, 50) -> (-34, 50) centre (-31.5, 50) ccw
  line L1 (-34, 5) -> (-34, 50)
  arc A1 (-34, 5) -> (-29, 5) centre (-31.5, 5) ccw
  line L2 (-19, 50) -> (-19, 5)
  arc A2 (-24, 5) -> (-19, 5) centre (-21.5, 5) ccw
  line L3 (-24, 5) -> (-24, 50)
  arc A3 (-19, 50) -> (-24, 50) centre (-21.5, 50) ccw
  arc A4 (1, 50) -> (-4, 50) centre (-1.5, 50) ccw
  line L4 (11, 50) -> (11, 5)
  arc A5 (6, 5) -> (11, 5) centre (8.5, 5) ccw
  line L5 (6, 5) -> (6, 50)
  arc A6 (11, 50) -> (6, 50) centre (8.5, 50) ccw
  line L6 (21, 50) -> (21, 5)
  arc A7 (16, 5) -> (21, 5) centre (18.5, 5) ccw
  line L7 (16, 5) -> (16, 50)
  arc A8 (21, 50) -> (16, 50) centre (18.5, 50) ccw
  line L8 (41, 50) -> (41, 5)
  arc A9 (36, 5) -> (41, 5) centre (38.5, 5) ccw
  line L9 (36, 5) -> (36, 50)
  arc A10 (41, 50) -> (36, 50) centre (38.5, 50) ccw
  line L10 (-29, -5) -> (-29, -50)
  arc A11 (-34, -50) -> (-29, -50) centre (-31.5, -50) ccw
  line L11 (-34, -50) -> (-34, -5)
  arc A12 (-29, -5) -> (-34, -5) centre (-31.5, -5) ccw
  line L12 (-17.3333, -5) -> (-17.3333, -50)
  arc A13 (-22.3333, -50) -> (-17.3333, -50) centre (-19.8333, -50) ccw
  line L13 (-22.3333, -50) -> (-22.3333, -5)
  arc A14 (-17.3333, -5) -> (-22.3333, -5) centre (-19.8333, -5) ccw
  line L14 (-5.6667, -5) -> (-5.6667, -50)
  arc A15 (-10.6667, -50) -> (-5.6667, -50) centre (-8.1667, -50) ccw
  line L15 (-10.6667, -50) -> (-10.6667, -5)
  arc A16 (-5.6667, -5) -> (-10.6667, -5) centre (-8.1667, -5) ccw
  line L16 (6, -5) -> (6, -50)
  arc A17 (1, -50) -> (6, -50) centre (3.5, -50) ccw
  line L17 (1, -50) -> (1, -5)
  arc A18 (6, -5) -> (1, -5) centre (3.5, -5) ccw
  line L18 (17.6667, -5) -> (17.6667, -50)
  arc A19 (12.6667, -50) -> (17.6667, -50) centre (15.1667, -50) ccw
  line L19 (12.6667, -50) -> (12.6667, -5)
  arc A20 (17.6667, -5) -> (12.6667, -5) centre (15.1667, -5) ccw
  line L20 (41, -5) -> (41, -50)
  arc A21 (36, -50) -> (41, -50) centre (38.5, -50) ccw
  line L21 (36, -50) -> (36, -5)
  arc A22 (41, -5) -> (36, -5) centre (38.5, -5) ccw
  dimension "d85" = 70
  dimension "d86" = 0
  dimension "d91" = 70
  dimension "d92" = 0
extrude "Extrude19" cut sketch "Sketch17" along normal blind 5 contours L0 A0 L1 A1 | L2 A2 L3 A3 | L4 A5 L5 A6 | L6 A7 L7 A8 | L8 A9 L9 A10 bodies 1
extrude "Extrude20" cut sketch "Sketch17" along normal blind 4 contours L10 A11 L11 A12 | L12 A13 L13 A14 | L14 A15 L15 A16 | L16 A17 L17 A18 | L18 A19 L19 A20 | L20 A21 L21 A22 bodies 1
hole "Hole1" at (-9.3669, 5.4726, 7) direction (0, 0, -1) diameter 2.529 depth 4 tip angle 118 bodies 3
thread "Thread1" "ISO Metric profile 3.0 M3x0.5 M3x0.5 6H" major diameter 3.086 minor diameter 2.529 pitch 0.5 angle 60 resizes the face on face at (-9.241, 4.2144, 4.3333) on bodies 3
hole "Hole2" at (-6.7121, 37.2637, 7) direction (0, 0, -1) diameter 2.529 depth 4 tip angle 118 bodies 4
thread "Thread2" "ISO Metric profile 3.0 M3x0.5 M3x0.5 6H" major diameter 3.086 minor diameter 2.529 pitch 0.5 angle 60 resizes the face on face at (-7.9762, 37.2952, 5.6667) on bodies 4
hole "Hole3" at (28.2811, 19.6527, 7) direction (0, 0, -1) diameter 2.529 depth 4 tip angle 118 bodies 6
thread "Thread3" "ISO Metric profile 3.0 M3x0.5 M3x0.5 6H" major diameter 3.086 minor diameter 2.529 pitch 0.5 angle 60 resizes the face on face at (28.407, 18.3945, 4.3333) on bodies 6
hole "Hole4" at (28.249, -42.7358, 7) direction (0, 0, -1) diameter 2.529 depth 4 tip angle 118 bodies 5
thread "Thread4" "ISO Metric profile 3.0 M3x0.5 M3x0.5 6H" major diameter 3.086 minor diameter 2.529 pitch 0.5 angle 60 resizes the face on face at (26.9849, -42.7043, 5.6667) on bodies 5
hole "Hole5" at (-36.2541, -58.894, 7) direction (0, 0, -1) diameter 2.529 depth 4 tip angle 118 bodies 7
thread "Thread5" "ISO Metric profile 3.0 M3x0.5 M3x0.5 6H" major diameter 3.086 minor diameter 2.529 pitch 0.5 angle 60 resizes the face on face at (-35.4906, -57.886, 5.6667) on bodies 7
combine "Combine1" operation add target body 2 tool bodies 1 7 6 4 3 5
fillet "Fillet1" radius 3 tangency weight 0.51671 6 edges at (-94.0003, -79, 0) (-180, -5, 0) (-61, 69, 0) (58, -0.7507, 0) (25.0001, -70.5015, 0) (-8.0002, -74.7507, 0) on bodies 2
fillet "Fillet2" radius 2 6 edges at (-13.9959, -68.7928, 2) (-73.498, -72.9826, 2) (19.012, -64.6029, 2) (52.0199, -0.8009, 2) (-173.9352, -4.9923, 2) (-60.9535, 62.9995, 2) on bodies 2
fillet "Fillet3" radius 2 1 edges at (-29.3384, 69, 15.8081) on bodies 2
fillet "Fillet4" radius 2 1 edges at (-29.3384, 63, 12.1919) on bodies 2
fillet "Fillet5" radius 2 1 edges at (58, 35, 29) on bodies 2
fillet "Fillet6" radius 2 1 edges at (52.0199, 35, 29) on bodies 2
fillet "Fillet7" radius 2 1 edges at (25.4296, -41.6423, 2) on bodies 2
fillet "Fillet8" radius 2 1 edges at (25.4617, 20.7462, 2) on bodies 2
fillet "Fillet9" radius 2 3 edges at (-12.1863, 6.5662, 2) (-9.5314, 38.3572, 2) (-39.0734, -57.8005, 2) on bodies 2
fillet "Fillet10" radius 2 1 edges at (-108, 40, 2) on bodies 2
fillet "Fillet11" radius 2 1 edges at (-108, 20, 2) on bodies 2
fillet "Fillet12" radius 2 1 edges at (-108, 25, 2) on bodies 2
fillet "Fillet13" radius 2 1 edges at (-108, 45, 2) on bodies 2
fillet "Fillet14" radius 1 4 edges at (4, -70.5015, 14) (4, -70.5015, 6) (-3, -70.5015, 10) (11, -70.5015, 10) on bodies 2
fillet "Fillet15" radius 0.5 4 edges at (21.6928, -70.5015, 11) (12.8347, -70.5015, 9.5) (21.6928, -70.5015, 8) (30.5509, -70.5015, 9.5) on bodies 2
sketch "Sketch19" plane through (0, 109.4985, 0) normal (0, -1, 0) x (1, 0, 0)
  line L0 (58, 43) -> (58, 45.5)
  line L1 (58, 45.5) -> (-98, 45.5)
  line L2 (-98, 45.5) -> (-98, 43)
  line L3 (-98, 43) -> (58, 43)
  line L4 (-6, 43) -> (-6, 45.5)
  dimension "d156" = 92
  constraint coincident L3 L4.start
  constraint coincident L1 L4.end
  constraint perpendicular L1 L4
  measures "d156" distance of L2 L4
extrude "Extrude21" add sketch "Sketch19" along normal blind 14.71 contours L1 L2 L3 L4 bodies 8
sketch "Sketch20" plane through (0, 0, 43) normal (0, 0, -1) x (1, 0, 0)
sketch "Sketch21" plane through (-98, 0, 0) normal (-1, 0, 0) x (0, -1, 0)
  line L0 (-241.95, 43) -> (-243.9167, 40.05)
  line L1 (-243.9167, 40.05) -> (-235.0833, 40.05)
  line L2 (-235.0833, 40.05) -> (-237.05, 43)
  line L3 (-237.05, 43) -> (-194.9089, 43)
  line L4 (-194.9089, 43) -> (-196.8422, 40.1)
  line L5 (-196.8422, 40.1) -> (-187.1667, 40.1)
  line L6 (-187.1667, 40.1) -> (-189.1, 43)
  line L7 (-189.1, 43) -> (-169.9, 43)
  line L8 (-169.9, 43) -> (-171.8333, 40.1)
  line L9 (-171.8333, 40.1) -> (-162.1667, 40.1)
  line L10 (-162.1667, 40.1) -> (-164.1, 43)
  line L11 (-164.1, 43) -> (-144.9, 43)
  line L12 (-144.9, 43) -> (-146.8333, 40.1)
  line L13 (-146.8333, 40.1) -> (-137.1667, 40.1)
  line L14 (-137.1667, 40.1) -> (-139.1, 43)
  line L15 (-139.1, 43) -> (-119.9, 43)
  line L16 (-119.9, 43) -> (-121.8333, 40.1)
  line L17 (-121.8333, 40.1) -> (-112.1667, 40.1)
  line L18 (-112.1667, 40.1) -> (-114.1, 43)
  line L19 (-114.1, 43) -> (-94.7885, 43)
  line L20 (-94.7885, 43) -> (-94.7885, 45.5)
  line L21 (-94.7885, 45.5) -> (-249, 45.5)
  line L22 (-249, 45.5) -> (-249, 43)
  line L23 (-249, 43) -> (-241.95, 43)
  line L24 (-94.7885, 43) -> (-249, 43)
  line L25 (-249, 43) -> (-249, 45.5)
  line L26 (-94.7885, 45.5) -> (-94.7885, 43)
  line L27 (-94.7885, 45.5) -> (-249, 45.5)
  constraint coincident L19.end L20.start
  constraint coincident L22.end L23.start
  constraint coincident L21.end L22.start
  constraint coincident L20.end L21.start
extrude "Extrude23" add 1 faces at (-98, 238.6833, 41.0333) along direction (-1, 0, 0) blind 85 on bodies 8 bodies 8
extrude "Extrude22" add sketch "Sketch21" along normal blind 8 contours L3 L7 L11 L15 L19 L20 L21 L22 L23 L24 L25 L26 L27 bodies 8
delete_face "DeleteFace1" 1 faces at (-69.4918, 43.3333, 6.5893) on bodies 2
delete_face "DeleteFace2" 1 faces at (-126.3333, 39.9977, 3.9048) on bodies 2
delete_face "DeleteFace3" 1 faces at (-89.6667, 40, 8) on bodies 2
delete_face "DeleteFace4" 1 faces at (-69.4918, 23.3333, 6.5893) on bodies 2
delete_face "DeleteFace5" 1 faces at (-126.3333, 19.9977, 3.9048) on bodies 2
delete_face "DeleteFace6" 1 faces at (-89.6667, 20, 8) on bodies 2
sketch "Sketch22" plane through (-183, 0, 0) normal (-1, 0, 0) x (0, -1, 0)
  line L0 (-241.95, 43) -> (-243.9167, 40.05)
  line L1 (-243.9167, 40.05) -> (-235.0833, 40.05)
  line L2 (-235.0833, 40.05) -> (-237.05, 43)
  line L3 (-237.05, 43) -> (-194.9089, 43)
  line L4 (-194.9089, 43) -> (-196.8422, 40.1)
  line L5 (-196.8422, 40.1) -> (-187.1667, 40.1)
  line L6 (-187.1667, 40.1) -> (-189.1, 43)
  line L7 (-189.1, 43) -> (-169.9, 43)
  line L8 (-169.9, 43) -> (-171.8333, 40.1)
  line L9 (-171.8333, 40.1) -> (-162.1667, 40.1)
  line L10 (-162.1667, 40.1) -> (-164.1, 43)
  line L11 (-164.1, 43) -> (-144.9, 43)
  line L12 (-144.9, 43) -> (-146.8333, 40.1)
  line L13 (-146.8333, 40.1) -> (-137.1667, 40.1)
  line L14 (-137.1667, 40.1) -> (-139.1, 43)
  line L15 (-139.1, 43) -> (-119.9, 43)
  line L16 (-119.9, 43) -> (-121.8333, 40.1)
  line L17 (-121.8333, 40.1) -> (-112.1667, 40.1)
  line L18 (-112.1667, 40.1) -> (-114.1, 43)
  line L19 (-114.1, 43) -> (-94.7885, 43)
  line L20 (-94.7885, 43) -> (-94.7885, 45.5)
  line L21 (-94.7885, 45.5) -> (-249, 45.5)
  line L22 (-249, 45.5) -> (-249, 43)
  line L23 (-249, 43) -> (-241.95, 43)
  line L24 (-119.9, 43) -> (-114.1, 43)
  line L25 (-114.1, 43) -> (-112.1667, 40.1)
  line L26 (-112.1667, 40.1) -> (-121.8333, 40.1)
  line L27 (-121.8333, 40.1) -> (-119.9, 43)
  line L28 (-139.1, 43) -> (-137.1667, 40.1)
  line L29 (-137.1667, 40.1) -> (-146.8333, 40.1)
  line L30 (-146.8333, 40.1) -> (-144.9, 43)
  line L31 (-144.9, 43) -> (-139.1, 43)
  line L32 (-164.1, 43) -> (-162.1667, 40.1)
  line L33 (-162.1667, 40.1) -> (-171.8333, 40.1)
  line L34 (-171.8333, 40.1) -> (-169.9, 43)
  line L35 (-169.9, 43) -> (-164.1, 43)
  line L36 (-189.1, 43) -> (-187.1667, 40.1)
  line L37 (-187.1667, 40.1) -> (-196.8422, 40.1)
  line L38 (-196.8422, 40.1) -> (-194.9089, 43)
  line L39 (-194.9089, 43) -> (-189.1, 43)
  line L40 (-237.05, 43) -> (-235.0833, 40.05)
  line L41 (-235.0833, 40.05) -> (-243.9167, 40.05)
  line L42 (-243.9167, 40.05) -> (-241.95, 43)
  line L43 (-241.95, 43) -> (-237.05, 43)
  constraint coincident L15.end L16.start
  constraint coincident L18.end L19.start
  constraint coincident L17.end L18.start
  constraint coincident L16.end L17.start
  constraint coincident L14.end L15.start
  constraint coincident L13.end L14.start
  constraint coincident L12.end L13.start
  constraint coincident L11.end L12.start
  constraint coincident L10.end L11.start
  constraint coincident L9.end L10.start
  constraint coincident L8.end L9.start
  constraint coincident L7.end L8.start
  constraint coincident L6.end L7.start
  constraint coincident L5.end L6.start
  constraint coincident L4.end L5.start
  constraint coincident L3.end L4.start
  constraint coincident L2.end L3.start
  constraint coincident L1.end L2.start
  constraint coincident L0.end L1.start
  constraint coincident L0.start L23.end
extrude "Extrude24" cut sketch "Sketch22" against normal blind 5 contours L0 L1 L2 L40 L41 L42 L43 | L4 L5 L6 L36 L37 L38 L39 | L8 L9 L10 L32 L33 L34 L35 | L16 L17 L18 L24 L25 L26 L27 | L12 L13 L14 L28 L29 L30 L31 bodies 8
extrude "Extrude25" cut 1 faces at (-183, 152.6295, 44.6667) along direction (1, 0, 0) blind 3 on bodies 8 bodies 8
extrude "Extrude26" cut 5 faces at (-178, 240.3167, 41.0333) (-178, 192.9726, 41.0667) (-178, 167.9667, 41.0667) (-178, 142.9667, 41.0667) (-178, 117.9667, 41.0667) along direction (1, 0, 0) blind 1 on bodies 8 bodies 8
sketch "Sketch23" plane through (58, 0, 0) normal (1, 0, 0) x (0, 1, 0)
  line L0 (62, 61) -> (64, 58)
  line L1 (64, 58) -> (55, 58)
  line L2 (55, 58) -> (57, 61)
  line L3 (57, 61) -> (62, 61)
  line L4 (15, 61) -> (9, 61)
  line L5 (9, 61) -> (7, 58)
  line L6 (7, 58) -> (17, 58)
  line L7 (17, 58) -> (15, 61)
  line L8 (-10, 61) -> (-8, 58)
  line L9 (-8, 58) -> (-18, 58)
  line L10 (-18, 58) -> (-16, 61)
  line L11 (-16, 61) -> (-10, 61)
  line L12 (-35, 61) -> (-33, 58)
  line L13 (-33, 58) -> (-43, 58)
  line L14 (-43, 58) -> (-41, 61)
  line L15 (-41, 61) -> (-35, 61)
  line L16 (-60, 61) -> (-58, 58)
  line L17 (-58, 58) -> (-68, 58)
  line L18 (-68, 58) -> (-66, 61)
  line L19 (-66, 61) -> (-60, 61)
  constraint horizontal L1
  constraint parallel L1 L3
  constraint parallel L3 L4
  constraint parallel L2 L5
  constraint parallel L4 L6
  constraint parallel L7 L8
  constraint parallel L4 L9
  constraint parallel L9 L11
  constraint parallel L8 L12
  constraint parallel L11 L13
  constraint parallel L13 L15
  constraint parallel L12 L16
  constraint parallel L15 L17
  constraint parallel L14 L18
  constraint parallel L17 L19
extrude "Extrude27" cut sketch "Sketch23" against normal blind 235 bodies 2
sketch "Sketch24" plane through (0, -72.9826, 0) normal (0, 1, 0) x (-1, 0, 0)
  line L0 (13.9959, 4) -> (133, 4)
  line L1 (133, 4) -> (133, 61)
  line L2 (133, 61) -> (132, 61)
  line L3 (132, 61) -> (132, 10)
  arc A0 (127, 10) -> (132, 10) centre (129.5, 10) ccw
  line L4 (127, 10) -> (127, 61)
  line L5 (127, 61) -> (124, 61)
  line L6 (124, 61) -> (124, 10)
  arc A1 (119, 10) -> (124, 10) centre (121.5, 10) ccw
  line L7 (119, 10) -> (119, 61)
  line L8 (119, 61) -> (116, 61)
  line L9 (116, 61) -> (116, 10)
  arc A2 (111, 10) -> (116, 10) centre (113.5, 10) ccw
  line L10 (111, 10) -> (111, 61)
  line L11 (111, 61) -> (108, 61)
  line L12 (108, 61) -> (108, 10)
  arc A3 (103, 10) -> (108, 10) centre (105.5, 10) ccw
  line L13 (103, 10) -> (103, 61)
  line L14 (103, 61) -> (100, 61)
  line L15 (100, 61) -> (100, 10)
  arc A4 (95, 10) -> (100, 10) centre (97.5, 10) ccw
  line L16 (95, 10) -> (95, 61)
  line L17 (95, 61) -> (13.9959, 61)
  line L18 (13.9959, 61) -> (13.9959, 4)
  line L19 (50, 61) -> (53, 61)
  line L20 (53, 61) -> (53, 0)
  line L21 (53, 0) -> (50, 0)
  line L22 (50, 0) -> (50, 61)
  constraint horizontal L19
  constraint vertical L20
  constraint horizontal L21
  constraint vertical L22
  constraint coincident L17 L19.start
extrude "Extrude28" add sketch "Sketch24" along normal blind 140 contours L0 L17 L19 L20 L22 bodies 2
extrude "Extrude29" add 1 faces at (-51, 17.6723, 4) along direction (0, 0, -1) blind 1 on bodies 2 bodies 2
extrude "Extrude30" cut 1 faces at (-53, 23.3333, 0.6667) along direction (-1, 0, 0) blind 2 on bodies 2 bodies 2
extrude "Extrude31" cut 1 faces at (-53, 43.3333, 0.6667) along direction (-1, 0, 0) blind 2 on bodies 2 bodies 2
extrude "Extrude32" add 1 faces at (-50, 23.3333, 0.6667) along direction (-1, 0, 0) blind 3 on bodies 2 bodies 2
extrude "Extrude33" add 1 faces at (-50, 43.3333, 0.6667) along direction (-1, 0, 0) blind 3 on bodies 2 bodies 2
extrude "Extrude34" cut 1 faces at (-55, 43.3333, 0.6667) along direction (-1, 0, 0) blind 1 on bodies 2 bodies 2
extrude "Extrude35" cut 1 faces at (-55, 23.3333, 0.6667) along direction (-1, 0, 0) blind 1 on bodies 2 bodies 2
extrude "Extrude36" add 3 faces at (-50, -66.6667, 0.6667) (-50, -51.6667, 0.6667) (-50, -36.6667, 0.6667) along direction (-1, 0, 0) blind 3 on bodies 2 bodies 2
extrude "Extrude37" add 3 faces at (-133, -36.6667, 0.6667) (-133, -51.6667, 0.6667) (-133, -66.6667, 0.6667) along direction (1, 0, 0) blind 77 on bodies 2 bodies 2
sketch "Sketch25" plane through (-95, 0, 0) normal (-1, 0, 0) x (0, -1, 0)
  line L0 (72.9826, 61) -> (72.9826, 10)
  line L1 (72.9826, 10) -> (79, 10)
  line L2 (79, 10) -> (79, 61)
  line L3 (79, 61) -> (72.9826, 61)
  line L4 (72.9826, 61) -> (79, 61)
  line L5 (79, 61) -> (79, 57)
  line L6 (79, 57) -> (72.9826, 57)
  line L7 (72.9826, 57) -> (72.9826, 61)
  constraint horizontal L4
  constraint vertical L5
  constraint horizontal L6
  constraint vertical L7
  constraint coincident L2 L5.end
  constraint coincident L0.start L3.end
extrude "Extrude38" add sketch "Sketch25" along normal blind 80 contours L0 L2 L3 L4 L5 L6 L7 bodies 2